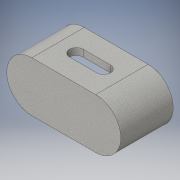
# Autodesk Inventor part: Concrete case
Saved by Autodesk Inventor 2016 SP2 (Build 200236200, 236)
## iProperties
Created: 2017-10-06
Part Number: Concrete case
Material: GFRC
Document SubType Name: Modeling
Designer: Jared
Density: 1.7 g/cm^3
Appearance: Flat - Polished Gray
Author: Jared
Autodesk Inventor part; units mm, degrees
ref_plane "YZ Plane" through (0, 0, 0) normal (1, 0, 0) x (0, 1, 0)
ref_plane "XZ Plane" through (0, 0, 0) normal (0, 1, 0) x (-1, 0, 0)
ref_plane "XY Plane" through (0, 0, 0) normal (0, 0, 1) x (1, 0, 0)
sketch "Sketch1" plane through (0, 0, 0) normal (0, 0, 1) x (1, 0, 0)
  line L0 (0, 0) -> (-177.8, 0) construction
  line L1 (0, 69.85) -> (-177.8, 69.85)
  line L2 (-177.8, -69.85) -> (0, -69.85)
  arc A0 (0, -69.85) -> (0, 69.85) centre (0, 0) ccw
  arc A1 (-177.8, 69.85) -> (-177.8, -69.85) centre (-177.8, 0) ccw
  point P0 (-88.9, 0)
  dimension "d0" = 177.8
  dimension "d1" = 139.7
  constraints: 8 end point, 4 point on circle, 4 tangent, 2 centre point, 1 horizontal, 1 midpoint, 1 parallel
  measures "d0" distance of L0.start L0.end
  measures "d1" diameter of A1
extrude "Extrusion1" add sketch "Sketch1" along normal blind 146.05
shell "Shell1" thickness 19.05 removed faces 1 at (-59.2667, -23.2833, 0)
sketch "Sketch2" plane through (-177.8, 69.85, 0) normal (0, 1, 0) x (1, 0, 0)
  line L0 (177.8, 0) -> (0, 0) projected
  line L1 (0, 0) -> (0, -146.05) projected
  line L2 (177.8, -146.05) -> (0, -146.05) projected
  line L3 (177.8, 0) -> (177.8, -146.05) projected
  line L4 (0, 0) -> (0, -146.05) projected
  line L5 (0, -73.025) -> (177.8, -73.025)
  line L6 (177.8, 0) -> (177.8, -127) projected
  line L7 (177.8, 0) -> (177.8, -146.05) projected
  line L8 (127, -73.025) -> (50.8, -73.025) construction
  line L9 (127, -53.975) -> (50.8, -53.975)
  line L10 (50.8, -92.075) -> (127, -92.075)
  arc A0 (127, -92.075) -> (127, -53.975) centre (127, -73.025) ccw
  arc A1 (50.8, -53.975) -> (50.8, -92.075) centre (50.8, -73.025) ccw
  point P0 (88.9, -73.025)
  dimension "d10" = 38.1
  dimension "d11" = 38.1
  constraints: 10 end point, 4 midpoint, 4 point on circle, 4 tangent, 2 centre point, 2 point on line, 1 parallel
  measures "d10" distance of point (88.9, -73.025) L8.end
  measures "d11" diameter of A1
extrude "Extrusion2" cut sketch "Sketch2" against normal up to surface (19.05 mm away) contours A0 L10 A1 L5 | L5 A1 L9 A0
body "Solid1"
